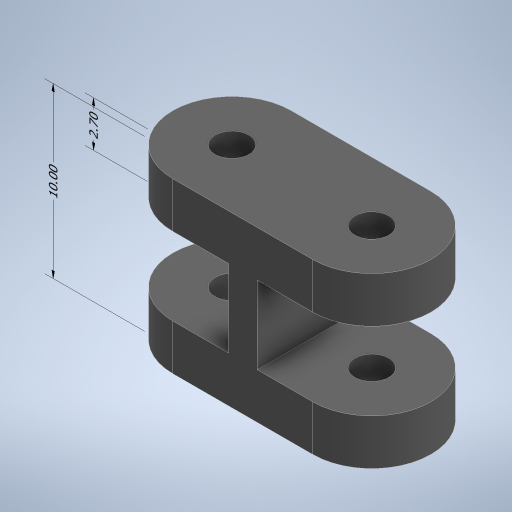
# Autodesk Inventor part: chain_1
Saved by Autodesk Inventor 2024.1 (Build 281209000, 209)
## iProperties
Created: 2025-01-18
Part Number: chain_1
Material: 一般
Document SubType Name: Modeling
Designer: hibik
Density: 1 g/cm^3
Appearance: 既定
Author: hibik
Autodesk Inventor part; units mm, degrees
ref_plane "YZ Plane" through (0, 0, 0) normal (1, 0, 0) x (0, 1, 0)
ref_plane "XZ Plane" through (0, 0, 0) normal (0, 1, 0) x (-1, 0, 0)
ref_plane "XY Plane" through (0, 0, 0) normal (0, 0, 1) x (1, 0, 0)
sketch "スケッチ1" plane through (0, 0, 0) normal (0, 1, 0) x (-1, 0, 0)
  circle A0 centre (0, 0) radius 1
  circle A1 centre (0, 0) radius 3.5
  circle A2 centre (-8.2843, 0) radius 3.5
  line L0 (0, -3.5) -> (-8.2843, -3.5)
  line L1 (-8.2843, -3.5) -> (-8.2843, 3.5) construction
  line L2 (-8.2843, 3.5) -> (0, 3.5)
  line L3 (0, 3.5) -> (0, -3.5) construction
  circle A3 centre (-8.2843, 0) radius 1
  line L4 (-3.2921, -3.5) -> (-4.9921, -3.5)
  line L5 (-4.9921, -3.5) -> (-4.9921, 3.5)
  line L6 (-4.9921, 3.5) -> (-3.2921, 3.5)
  line L7 (-3.2921, 3.5) -> (-3.2921, -3.5)
  circle A4 centre (-4.1421, 10) radius 10
  line L8 (0, 0) -> (-8.2843, 0)
  line L9 (-4.1421, 10) -> (0, 0)
  line L10 (-4.1421, 10) -> (-8.2843, 0)
  line L11 (-4.1421, -3.5) -> (-4.1421, 3.5) construction
  point P0 (-8.2843, -3.5)
  point P1 (-3.2921, 3.5)
  point P2 (-4.1421, 0)
  dimension "d1" = 7
  dimension "d0" = 2
  dimension "d13" = 20
  dimension "d14" = 45
  dimension "d31" = 1.7
  constraints: 24 end point, 4 coincident, 4 horizontal, 4 midpoint, 4 parallel, 3 centre point, 3 perpendicular, 2 point on line, 1 equal radius, 1 horizontal alignment, 1 tangent, 1 vertical alignment, 6 other
  measures "d0" diameter of A0
  measures "d13" diameter of A4
  measures "d14" angle of L10 L9
  measures "d31" distance between parallel lines of L5 L7
extrude "押し出し3" add sketch "スケッチ1" along normal blind 5 contours A0 A4 A1 L7 L8 | A0 L9 A1 A4 | L8 L7 A4 A0 | A0 A4 L7 A1 L9 | L8 A1 A4 L7 | L7 A1 L8 | L9 L2 A1 | A1 L7 L2 L9 | A4 A1 L7 | L7 L0 L5 A2 L8 A1 | A1 L0 L7 | L8 A4 A1 | A1 A4 A2 L5 L2 L7 | A4 A3 L8 L5 A2 | A2 L10 A3 A4 | L8 A2 A4 | L2 L10 A2 | A2 L5 L0 | A4 L5 A2 | A2 L8 L5 A4 | A2 L5 L8 | L5 A2 L10 L2 | A2 L5 A4 A3 L10 | A3 A4 L5 L8
extrude "押し出し4" cut sketch "スケッチ1" along normal blind 2.3 contours A0 A4 A1 L7 L8 | A0 L9 A1 A4 | L8 L7 A4 A0 | A0 A4 L7 A1 L9 | L9 L2 A1 | A1 L7 L2 L9 | A1 L0 L7 | A4 A3 L8 L5 A2 | A2 L10 A3 A4 | L2 L10 A2 | A2 L5 L0 | L5 A2 L10 L2 | A2 L5 A4 A3 L10 | A3 A4 L5 L8
mirror "ミラー2" about plane through (4.1421, 0, 0) normal (0, -1, 0)
